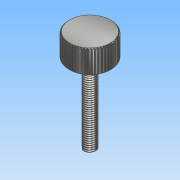
# Autodesk Inventor part: Регулировочный винт
Saved by Autodesk Inventor 2017 (Build 210142000, 142)
## iProperties
Part Number: Регулировочный винт
Material: Типовые
Document SubType Name: Modeling
Designer: STALKER
Density: 1 g/cm^3
Appearance: Сталь — полированная
Author: STALKER
Autodesk Inventor part; units mm, degrees
ref_plane "YZ Plane" through (0, 0, 0) normal (1, 0, 0) x (0, 1, 0)
ref_plane "XZ Plane" through (0, 0, 0) normal (0, 1, 0) x (-1, 0, 0)
ref_plane "XY Plane" through (0, 0, 0) normal (0, 0, 1) x (1, 0, 0)
sketch "Эскиз1" plane through (0, 0, 0) normal (0, 0, 1) x (1, 0, 0)
  circle A0 centre (0, 0) radius 5.5
  circle A1 centre (0, 0) radius 1.5
  dimension "d0" = 11
  dimension "d1" = 3
  constraints: 2 centre point, 2 coincident
  measures "d0" diameter of A0
  measures "d1" diameter of A1
extrude "Выдавливание1" add sketch "Эскиз1" along normal blind 6 contours A0 | A1
extrude "Выдавливание2" add sketch "Эскиз1" against normal blind 20 contours A1
thread "Резьба1" size "M3x0.5" class "6g" standard "ANSI Metric M Profile" full length
sketch "Эскиз3" plane through (0, 0, -20) normal (1, 0, 0) x (0, 1, 0)
  line L0 (1.5, 0) -> (1.5, 20)
  line L1 (1.5, 20) -> (1.1293, 20)
  line L2 (1.1293, 20) -> (1.1293, 0)
  line L3 (1.1293, 0) -> (1.5, 0)
  line L4 (0, -5.8544) -> (0, 31.3091) projected
  constraints: 8 end point
revolve "Вращение1" cut sketch "Эскиз3" angle 360 about axis through (0, 0, -20) along (0, 0, 1)
sketch "Эскиз4" plane through (0, 0, -20) normal (1, 0, 0) x (0, 1, 0)
  line L0 (1.5, 0) -> (1.5, 20)
  line L1 (1.5, 20) -> (1.1293, 20)
  line L2 (1.1293, 20) -> (1.1293, 0)
  line L3 (1.1293, 0) -> (1.5, 0)
  line L4 (0, -5.8544) -> (0, 31.3091) projected
  constraints: 8 end point
revolve "Вращение2" add sketch "Эскиз4" angle 360 about axis through (0, 0, -20) along (0, 0, 1) separate body
sketch "Эскиз2" plane through (0, 0, -20) normal (-1, 0, 0) x (0, 0, 1)
  line L0 (-0.2918, -1.1547) -> (-0.2501, -1.1547) construction
  line L1 (0.0416, -1.4749) -> (-0.0001, -1.5549) construction
  line L2 (-0.5001, -1.5549) -> (-0.5418, -1.4749) construction
  line L3 (-0.2084, -1.1547) -> (-0.2501, -1.0747) construction
  line L4 (-0.2501, -1.0747) -> (-0.2918, -1.1547) construction
  line L5 (-0.5001, -1.5549) -> (-0.4584, -1.4749) construction
  line L6 (-0.2084, -1.1547) -> (-0.0418, -1.4749)
  line L7 (-0.5418, -1.4749) -> (-0.4584, -1.4749) construction
  arc A0 (-0.5418, -1.4749) -> (-0.5001, -1.5002) centre (-0.5001, -1.4532) ccw construction
  line L8 (0.0416, -1.4749) -> (-0.0418, -1.4749) construction
  line L9 (-0.5001, -1.5549) -> (-0.5001, -1.4749) construction
  line L10 (-0.0001, -1.5549) -> (-0.0001, -1.4749) construction
  line L11 (-0.2501, -1.0747) -> (-0.2501, -1.1294) construction
  line L12 (-0.5001, -1.5002) -> (-0.0001, -1.5002)
  arc A1 (-0.5001, -1.5002) -> (-0.4584, -1.4749) centre (-0.5001, -1.4532) ccw
  line L13 (-0.0418, -1.4749) -> (-0.0001, -1.5549) construction
  line L14 (-0.4584, -1.4749) -> (-0.2918, -1.1547)
  line L15 (-0.0001, -0.0002) -> (-0.0001, 0.0177)
  line L16 (-0.0001, 0.0177) -> (-0.0001, -0.0002)
  line L17 (-0.0001, -0.0002) -> (0.0334, -0.0002)
  arc A2 (-0.0418, -1.4749) -> (-0.0001, -1.5002) centre (-0.0001, -1.4532) ccw
  arc A3 (-0.0001, -1.5002) -> (0.0416, -1.4749) centre (-0.0001, -1.4532) ccw construction
  arc A4 (-0.2501, -1.1294) -> (-0.2918, -1.1547) centre (-0.2501, -1.1764) ccw
  arc A5 (-0.2084, -1.1547) -> (-0.2501, -1.1294) centre (-0.2501, -1.1764) ccw
  line L18 (-0.2501, -1.1294) -> (-0.2501, -1.1547) construction
  line L19 (-0.2501, -1.1547) -> (-0.2084, -1.1547) construction
  dimension "d8" = 55
  dimension "d9" = 0.08
  dimension "d10" = 0.08
  dimension "Эскиз2_ThreadOffset" = 0
  dimension "Эскиз2_MajorRadius" = 1.5
  dimension "d13" = 0.5
  dimension "Эскиз2_MinorRadius" = 1.1293
  constraints: 40 end point, 12 point on circle, 10 parallel, 8 tangent, 6 centre point, 6 collinear, 2 midpoint, 2 point on line, 1 horizontal, 1 perpendicular, 3 other
  measures "d8" angle of L6 L14
  measures "d9" distance of L3.end L0.end
  measures "d10" distance of L1.end L10.end
  measures "Эскиз2_ThreadOffset" distance between parallel lines of L15 L10
  measures "Эскиз2_MajorRadius" distance from line of L12 L15.start
  measures "d13" distance from line of L1.end L9
  measures "Эскиз2_MinorRadius" distance edge to line of A5 L17
coil "Пружина1" sketch "Эскиз2" operation cut axis through (0, 0, -20) along (0, 0, 1) pitch 0.5005 turns 41.958042 hand right bodies 2
chamfer "Фаска1" distance 0.3 angle 45 2 edges at (-5.5, 0, 0) (-5.5, 0, 6)
sketch "Эскиз5" plane through (0, 0, 6) normal (0, 0, 1) x (1, 0, 0)
  line L0 (0, 0) -> (0, 10.4) construction
  line L1 (-0.525, 5.6749) -> (0, 5.2)
  line L2 (0, 5.2) -> (0.525, 5.6749)
  line L3 (0.525, 5.6749) -> (-0.525, 5.6749)
  circle A0 centre (0, 0) radius 5.2 projected
  dimension "d30" = 1.05
  constraints: 8 end point, 1 horizontal, 1 midpoint, 1 vertical alignment, 2 other
  measures "d30" distance of L2.end L1.start
extrude "Выдавливание3" cut sketch "Эскиз5" against normal blind 20 contours L3 L2 L1 bodies 1
pattern_circular "Круговой массив1" count 54 over 360 about axis through (0, 0, 0) along (0, 0, 1) of "Выдавливание3" bodies 1
equation "\"d8\" = d15"
equation "\"d9\" = 0.160083 * Эскиз2_Pitch"
equation "\"d10\" = 0.160083 * Эскиз2_Pitch"
equation "\"d13\" = Эскиз2_Pitch"
equation "\"d15\" = 55deg"
equation "\"Эскиз2_Pitch\" = 0.5"
